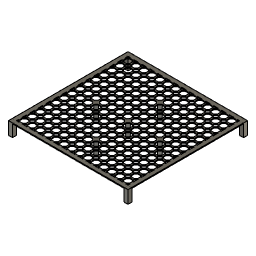
anticoprophagia mouse bedding (Autodesk Fusion 360 design; units mm, degrees)
Autodesk Fusion 360 part; units mm, degrees
(part 1 of 6)
sketch "Sketch1" plane through (0, 0, 0) normal (0, 0, 1) x (1, 0, 0)
  line L0 (-75, -75) -> (75, -75)
  line L1 (75, -75) -> (75, 75)
  line L2 (75, 75) -> (-75, 75)
  line L3 (-75, 75) -> (-75, -75)
  line L4 (-75, -75) -> (75, 75) construction
  line L5 (75, -75) -> (-75, 75) construction
  line L6 (-70, 70) -> (70, 70)
  line L7 (70, 70) -> (70, -70)
  line L8 (70, -70) -> (-70, -70)
  line L9 (-70, -70) -> (-70, 70)
  line L10 (-70, 70) -> (70, -70) construction
  line L11 (70, 70) -> (-70, -70) construction
  line L12 (-70, 70) -> (-60, 70)
  line L13 (-62.9289, 60) -> (-60, 62.9289)
  line L14 (-60, 62.9289) -> (-60, 67.0711)
  line L15 (-60, 67.0711) -> (-62.9289, 70)
  line L16 (-62.9289, 70) -> (-67.0711, 70)
  line L17 (-67.0711, 70) -> (-70, 67.0711)
  line L18 (-70, 67.0711) -> (-70, 62.9289)
  line L19 (-70, 62.9289) -> (-67.0711, 60)
  line L20 (-67.0711, 60) -> (-62.9289, 60)
  line L21 (-61, 63.3431) -> (-61, 66.6569)
  line L22 (-61, 66.6569) -> (-63.3431, 69)
  line L23 (-63.3431, 69) -> (-66.6569, 69)
  line L24 (-66.6569, 69) -> (-69, 66.6569)
  line L25 (-69, 66.6569) -> (-69, 63.3431)
  line L26 (-69, 63.3431) -> (-66.6569, 61)
  line L27 (-66.6569, 61) -> (-63.3431, 61)
  line L28 (-63.3431, 61) -> (-61, 63.3431)
  line L29 (-60, 67.0711) -> (-60, 62.9289)
  line L30 (-57.0711, 70) -> (-60, 67.0711)
  line L31 (-56.6569, 69) -> (-59, 66.6569)
  line L32 (-53.3431, 69) -> (-56.6569, 69)
  line L33 (-51, 66.6569) -> (-53.3431, 69)
  line L34 (-51, 63.3431) -> (-51, 66.6569)
  line L35 (-53.3431, 61) -> (-51, 63.3431)
  line L36 (-56.6569, 61) -> (-53.3431, 61)
  line L37 (-59, 63.3431) -> (-56.6569, 61)
  line L38 (-59, 66.6569) -> (-59, 63.3431)
  line L39 (-60, 62.9289) -> (-57.0711, 60)
  line L40 (-57.0711, 60) -> (-52.9289, 60)
  line L41 (-52.9289, 60) -> (-50, 62.9289)
  line L42 (-50, 62.9289) -> (-50, 67.0711)
  line L43 (-50, 67.0711) -> (-52.9289, 70)
  line L44 (-50, 67.0711) -> (-50, 62.9289)
  line L45 (-47.0711, 70) -> (-50, 67.0711)
  line L46 (-46.6569, 69) -> (-49, 66.6569)
  line L47 (-43.3431, 69) -> (-46.6569, 69)
  line L48 (-41, 66.6569) -> (-43.3431, 69)
  line L49 (-41, 63.3431) -> (-41, 66.6569)
  line L50 (-43.3431, 61) -> (-41, 63.3431)
  line L51 (-46.6569, 61) -> (-43.3431, 61)
  line L52 (-49, 63.3431) -> (-46.6569, 61)
  line L53 (-49, 66.6569) -> (-49, 63.3431)
  line L54 (-50, 62.9289) -> (-47.0711, 60)
  line L55 (-47.0711, 60) -> (-42.9289, 60)
  line L56 (-42.9289, 60) -> (-40, 62.9289)
  line L57 (-40, 62.9289) -> (-40, 67.0711)
  line L58 (-40, 67.0711) -> (-42.9289, 70)
  line L59 (-40, 67.0711) -> (-40, 62.9289)
  line L60 (-37.0711, 70) -> (-40, 67.0711)
  line L61 (-36.6569, 69) -> (-39, 66.6569)
  line L62 (-33.3431, 69) -> (-36.6569, 69)
  line L63 (-31, 66.6569) -> (-33.3431, 69)
  line L64 (-31, 63.3431) -> (-31, 66.6569)
  line L65 (-33.3431, 61) -> (-31, 63.3431)
  line L66 (-36.6569, 61) -> (-33.3431, 61)
  line L67 (-39, 63.3431) -> (-36.6569, 61)
  line L68 (-39, 66.6569) -> (-39, 63.3431)
  line L69 (-40, 62.9289) -> (-37.0711, 60)
  line L70 (-37.0711, 60) -> (-32.9289, 60)
  line L71 (-32.9289, 60) -> (-30, 62.9289)
  line L72 (-30, 62.9289) -> (-30, 67.0711)
  line L73 (-30, 67.0711) -> (-32.9289, 70)
  line L74 (-30, 67.0711) -> (-30, 62.9289)
  line L75 (-27.0711, 70) -> (-30, 67.0711)
  line L76 (-26.6569, 69) -> (-29, 66.6569)
  line L77 (-23.3431, 69) -> (-26.6569, 69)
  line L78 (-21, 66.6569) -> (-23.3431, 69)
  line L79 (-21, 63.3431) -> (-21, 66.6569)
  line L80 (-23.3431, 61) -> (-21, 63.3431)
  line L81 (-26.6569, 61) -> (-23.3431, 61)
  line L82 (-29, 63.3431) -> (-26.6569, 61)
  line L83 (-29, 66.6569) -> (-29, 63.3431)
  line L84 (-30, 62.9289) -> (-27.0711, 60)
  line L85 (-27.0711, 60) -> (-22.9289, 60)
  line L86 (-22.9289, 60) -> (-20, 62.9289)
  line L87 (-20, 62.9289) -> (-20, 67.0711)
  line L88 (-20, 67.0711) -> (-22.9289, 70)
  line L89 (-20, 67.0711) -> (-20, 62.9289)
  line L90 (-17.0711, 70) -> (-20, 67.0711)
  line L91 (-16.6569, 69) -> (-19, 66.6569)
  line L92 (-13.3431, 69) -> (-16.6569, 69)
  line L93 (-11, 66.6569) -> (-13.3431, 69)
  line L94 (-11, 63.3431) -> (-11, 66.6569)
  line L95 (-13.3431, 61) -> (-11, 63.3431)
  line L96 (-16.6569, 61) -> (-13.3431, 61)
  line L97 (-19, 63.3431) -> (-16.6569, 61)
  line L98 (-19, 66.6569) -> (-19, 63.3431)
  line L99 (-20, 62.9289) -> (-17.0711, 60)
  line L100 (-17.0711, 60) -> (-12.9289, 60)
  line L101 (-12.9289, 60) -> (-10, 62.9289)
  line L102 (-10, 62.9289) -> (-10, 67.0711)
  line L103 (-10, 67.0711) -> (-12.9289, 70)
  line L104 (-10, 67.0711) -> (-10, 62.9289)
  line L105 (-7.0711, 70) -> (-10, 67.0711)
  line L106 (-6.6569, 69) -> (-9, 66.6569)
  line L107 (-3.3431, 69) -> (-6.6569, 69)
  line L108 (-1, 66.6569) -> (-3.3431, 69)
  line L109 (-1, 63.3431) -> (-1, 66.6569)
  line L110 (-3.3431, 61) -> (-1, 63.3431)
  line L111 (-6.6569, 61) -> (-3.3431, 61)
  line L112 (-9, 63.3431) -> (-6.6569, 61)
  line L113 (-9, 66.6569) -> (-9, 63.3431)
  line L114 (-10, 62.9289) -> (-7.0711, 60)
  line L115 (-7.0711, 60) -> (-2.9289, 60)
  line L116 (-2.9289, 60) -> (0, 62.9289)
  line L117 (0, 62.9289) -> (0, 67.0711)
  line L118 (0, 67.0711) -> (-2.9289, 70)
  line L119 (0, 67.0711) -> (0, 62.9289)
  line L120 (2.9289, 70) -> (0, 67.0711)
  line L121 (3.3431, 69) -> (1, 66.6569)
  line L122 (6.6569, 69) -> (3.3431, 69)
  line L123 (9, 66.6569) -> (6.6569, 69)
  line L124 (9, 63.3431) -> (9, 66.6569)
  line L125 (6.6569, 61) -> (9, 63.3431)
  line L126 (3.3431, 61) -> (6.6569, 61)
  line L127 (1, 63.3431) -> (3.3431, 61)
  line L128 (1, 66.6569) -> (1, 63.3431)
  line L129 (0, 62.9289) -> (2.9289, 60)
  line L130 (2.9289, 60) -> (7.0711, 60)
  line L131 (7.0711, 60) -> (10, 62.9289)
  line L132 (10, 62.9289) -> (10, 67.0711)
  line L133 (10, 67.0711) -> (7.0711, 70)
  line L134 (10, 67.0711) -> (10, 62.9289)
  line L135 (12.9289, 70) -> (10, 67.0711)
  line L136 (13.3431, 69) -> (11, 66.6569)
  line L137 (16.6569, 69) -> (13.3431, 69)
  line L138 (19, 66.6569) -> (16.6569, 69)
  line L139 (19, 63.3431) -> (19, 66.6569)
  line L140 (16.6569, 61) -> (19, 63.3431)
  line L141 (13.3431, 61) -> (16.6569, 61)
  line L142 (11, 63.3431) -> (13.3431, 61)
  line L143 (11, 66.6569) -> (11, 63.3431)
  line L144 (10, 62.9289) -> (12.9289, 60)
  line L145 (12.9289, 60) -> (17.0711, 60)
  line L146 (17.0711, 60) -> (20, 62.9289)
  line L147 (20, 62.9289) -> (20, 67.0711)
  line L148 (20, 67.0711) -> (17.0711, 70)
  line L149 (20, 67.0711) -> (20, 62.9289)
  line L150 (22.9289, 70) -> (20, 67.0711)
  line L151 (23.3431, 69) -> (21, 66.6569)
  line L152 (26.6569, 69) -> (23.3431, 69)
  line L153 (29, 66.6569) -> (26.6569, 69)
  line L154 (29, 63.3431) -> (29, 66.6569)
  line L155 (26.6569, 61) -> (29, 63.3431)
  line L156 (23.3431, 61) -> (26.6569, 61)
  line L157 (21, 63.3431) -> (23.3431, 61)
  line L158 (21, 66.6569) -> (21, 63.3431)
  line L159 (20, 62.9289) -> (22.9289, 60)
  line L160 (22.9289, 60) -> (27.0711, 60)
  line L161 (27.0711, 60) -> (30, 62.9289)
  line L162 (30, 62.9289) -> (30, 67.0711)
  line L163 (30, 67.0711) -> (27.0711, 70)
  line L164 (30, 67.0711) -> (30, 62.9289)
  line L165 (32.9289, 70) -> (30, 67.0711)
  line L166 (33.3431, 69) -> (31, 66.6569)
  line L167 (36.6569, 69) -> (33.3431, 69)
  line L168 (39, 66.6569) -> (36.6569, 69)
  line L169 (39, 63.3431) -> (39, 66.6569)
  line L170 (36.6569, 61) -> (39, 63.3431)
  line L171 (33.3431, 61) -> (36.6569, 61)
  line L172 (31, 63.3431) -> (33.3431, 61)
  line L173 (31, 66.6569) -> (31, 63.3431)
  line L174 (30, 62.9289) -> (32.9289, 60)
  line L175 (32.9289, 60) -> (37.0711, 60)
  line L176 (37.0711, 60) -> (40, 62.9289)
  line L177 (40, 62.9289) -> (40, 67.0711)
  line L178 (40, 67.0711) -> (37.0711, 70)
  line L179 (40, 67.0711) -> (40, 62.9289)
  line L180 (42.9289, 70) -> (40, 67.0711)
  line L181 (43.3431, 69) -> (41, 66.6569)
  line L182 (46.6569, 69) -> (43.3431, 69)
  line L183 (49, 66.6569) -> (46.6569, 69)
  line L184 (49, 63.3431) -> (49, 66.6569)
  line L185 (46.6569, 61) -> (49, 63.3431)
  line L186 (43.3431, 61) -> (46.6569, 61)
  line L187 (41, 63.3431) -> (43.3431, 61)
  line L188 (41, 66.6569) -> (41, 63.3431)
  line L189 (40, 62.9289) -> (42.9289, 60)
  line L190 (42.9289, 60) -> (47.0711, 60)
  line L191 (47.0711, 60) -> (50, 62.9289)
  line L192 (50, 62.9289) -> (50, 67.0711)
  line L193 (50, 67.0711) -> (47.0711, 70)
  line L194 (50, 67.0711) -> (50, 62.9289)
  line L195 (52.9289, 70) -> (50, 67.0711)
  line L196 (53.3431, 69) -> (51, 66.6569)
  line L197 (56.6569, 69) -> (53.3431, 69)
  line L198 (59, 66.6569) -> (56.6569, 69)
  line L199 (59, 63.3431) -> (59, 66.6569)
  line L200 (56.6569, 61) -> (59, 63.3431)
  line L201 (53.3431, 61) -> (56.6569, 61)
  line L202 (51, 63.3431) -> (53.3431, 61)
  line L203 (51, 66.6569) -> (51, 63.3431)
  line L204 (50, 62.9289) -> (52.9289, 60)
  line L205 (52.9289, 60) -> (57.0711, 60)
  line L206 (57.0711, 60) -> (60, 62.9289)
  line L207 (60, 62.9289) -> (60, 67.0711)
  line L208 (60, 67.0711) -> (57.0711, 70)
  line L209 (60, 67.0711) -> (60, 62.9289)
  line L210 (62.9289, 70) -> (60, 67.0711)
  line L211 (63.3431, 69) -> (61, 66.6569)
  line L212 (66.6569, 69) -> (63.3431, 69)
  line L213 (69, 66.6569) -> (66.6569, 69)
  line L214 (69, 63.3431) -> (69, 66.6569)
  line L215 (66.6569, 61) -> (69, 63.3431)
  line L216 (63.3431, 61) -> (66.6569, 61)
  line L217 (61, 63.3431) -> (63.3431, 61)
  line L218 (61, 66.6569) -> (61, 63.3431)
  line L219 (60, 62.9289) -> (62.9289, 60)
  line L220 (62.9289, 60) -> (67.0711, 60)
  line L221 (67.0711, 60) -> (70, 62.9289)
  line L222 (70, 62.9289) -> (70, 67.0711)
  line L223 (70, 67.0711) -> (67.0711, 70)
  line L224 (-70, 57.0711) -> (-70, 52.9289)
  line L225 (-67.0711, 60) -> (-70, 57.0711)
  line L226 (-66.6569, 59) -> (-69, 56.6569)
  line L227 (-63.3431, 59) -> (-66.6569, 59)
  line L228 (-61, 56.6569) -> (-63.3431, 59)
  line L229 (-61, 53.3431) -> (-61, 56.6569)
  line L230 (-63.3431, 51) -> (-61, 53.3431)
  line L231 (-66.6569, 51) -> (-63.3431, 51)
  line L232 (-69, 53.3431) -> (-66.6569, 51)
  line L233 (-69, 56.6569) -> (-69, 53.3431)
  line L234 (-70, 52.9289) -> (-67.0711, 50)
  line L235 (-67.0711, 50) -> (-62.9289, 50)
  line L236 (-62.9289, 50) -> (-60, 52.9289)
  line L237 (-60, 52.9289) -> (-60, 57.0711)
  line L238 (-60, 57.0711) -> (-62.9289, 60)
  line L239 (-60, 57.0711) -> (-60, 52.9289)
  line L240 (-57.0711, 60) -> (-60, 57.0711)
  line L241 (-56.6569, 59) -> (-59, 56.6569)
  line L242 (-53.3431, 59) -> (-56.6569, 59)
  line L243 (-51, 56.6569) -> (-53.3431, 59)
  line L244 (-51, 53.3431) -> (-51, 56.6569)
  line L245 (-53.3431, 51) -> (-51, 53.3431)
  line L246 (-56.6569, 51) -> (-53.3431, 51)
  line L247 (-59, 53.3431) -> (-56.6569, 51)
  line L248 (-59, 56.6569) -> (-59, 53.3431)
  line L249 (-60, 52.9289) -> (-57.0711, 50)
  line L250 (-57.0711, 50) -> (-52.9289, 50)
  line L251 (-52.9289, 50) -> (-50, 52.9289)
  line L252 (-50, 52.9289) -> (-50, 57.0711)
  line L253 (-50, 57.0711) -> (-52.9289, 60)
  line L254 (-50, 57.0711) -> (-50, 52.9289)
  line L255 (-47.0711, 60) -> (-50, 57.0711)
  line L256 (-46.6569, 59) -> (-49, 56.6569)
  line L257 (-43.3431, 59) -> (-46.6569, 59)
  line L258 (-41, 56.6569) -> (-43.3431, 59)
  line L259 (-41, 53.3431) -> (-41, 56.6569)
  line L260 (-43.3431, 51) -> (-41, 53.3431)
  line L261 (-46.6569, 51) -> (-43.3431, 51)
  line L262 (-49, 53.3431) -> (-46.6569, 51)
  line L263 (-49, 56.6569) -> (-49, 53.3431)
  line L264 (-50, 52.9289) -> (-47.0711, 50)
  line L265 (-47.0711, 50) -> (-42.9289, 50)
  line L266 (-42.9289, 50) -> (-40, 52.9289)
  line L267 (-40, 52.9289) -> (-40, 57.0711)
  line L268 (-40, 57.0711) -> (-42.9289, 60)
  line L269 (-40, 57.0711) -> (-40, 52.9289)
  line L270 (-37.0711, 60) -> (-40, 57.0711)
  line L271 (-36.6569, 59) -> (-39, 56.6569)
  line L272 (-33.3431, 59) -> (-36.6569, 59)
  line L273 (-31, 56.6569) -> (-33.3431, 59)
  line L274 (-31, 53.3431) -> (-31, 56.6569)
  line L275 (-33.3431, 51) -> (-31, 53.3431)
  line L276 (-36.6569, 51) -> (-33.3431, 51)
  line L277 (-39, 53.3431) -> (-36.6569, 51)
  line L278 (-39, 56.6569) -> (-39, 53.3431)
  line L279 (-40, 52.9289) -> (-37.0711, 50)
  line L280 (-37.0711, 50) -> (-32.9289, 50)
  line L281 (-32.9289, 50) -> (-30, 52.9289)
  line L282 (-30, 52.9289) -> (-30, 57.0711)
  line L283 (-30, 57.0711) -> (-32.9289, 60)
  line L284 (-30, 57.0711) -> (-30, 52.9289)
  line L285 (-27.0711, 60) -> (-30, 57.0711)
  line L286 (-26.6569, 59) -> (-29, 56.6569)
  line L287 (-23.3431, 59) -> (-26.6569, 59)
  line L288 (-21, 56.6569) -> (-23.3431, 59)
  line L289 (-21, 53.3431) -> (-21, 56.6569)
  line L290 (-23.3431, 51) -> (-21, 53.3431)
  line L291 (-26.6569, 51) -> (-23.3431, 51)
  line L292 (-29, 53.3431) -> (-26.6569, 51)
  line L293 (-29, 56.6569) -> (-29, 53.3431)
  line L294 (-30, 52.9289) -> (-27.0711, 50)
  line L295 (-27.0711, 50) -> (-22.9289, 50)
  line L296 (-22.9289, 50) -> (-20, 52.9289)
  line L297 (-20, 52.9289) -> (-20, 57.0711)
  line L298 (-20, 57.0711) -> (-22.9289, 60)
  line L299 (-20, 57.0711) -> (-20, 52.9289)
  line L300 (-17.0711, 60) -> (-20, 57.0711)
  line L301 (-16.6569, 59) -> (-19, 56.6569)
  line L302 (-13.3431, 59) -> (-16.6569, 59)
  line L303 (-11, 56.6569) -> (-13.3431, 59)
  line L304 (-11, 53.3431) -> (-11, 56.6569)
  line L305 (-13.3431, 51) -> (-11, 53.3431)
  line L306 (-16.6569, 51) -> (-13.3431, 51)
  line L307 (-19, 53.3431) -> (-16.6569, 51)
  line L308 (-19, 56.6569) -> (-19, 53.3431)
  line L309 (-20, 52.9289) -> (-17.0711, 50)
  line L310 (-17.0711, 50) -> (-12.9289, 50)
  line L311 (-12.9289, 50) -> (-10, 52.9289)
  line L312 (-10, 52.9289) -> (-10, 57.0711)
  line L313 (-10, 57.0711) -> (-12.9289, 60)
  line L314 (-10, 57.0711) -> (-10, 52.9289)
  line L315 (-7.0711, 60) -> (-10, 57.0711)
  line L316 (-6.6569, 59) -> (-9, 56.6569)
  line L317 (-3.3431, 59) -> (-6.6569, 59)
  line L318 (-1, 56.6569) -> (-3.3431, 59)
  line L319 (-1, 53.3431) -> (-1, 56.6569)
  line L320 (-3.3431, 51) -> (-1, 53.3431)
  line L321 (-6.6569, 51) -> (-3.3431, 51)
  line L322 (-9, 53.3431) -> (-6.6569, 51)
  line L323 (-9, 56.6569) -> (-9, 53.3431)
  line L324 (-10, 52.9289) -> (-7.0711, 50)
  line L325 (-7.0711, 50) -> (-2.9289, 50)
  line L326 (-2.9289, 50) -> (0, 52.9289)
  line L327 (0, 52.9289) -> (0, 57.0711)
  line L328 (0, 57.0711) -> (-2.9289, 60)
  line L329 (0, 57.0711) -> (0, 52.9289)
  line L330 (2.9289, 60) -> (0, 57.0711)
  line L331 (3.3431, 59) -> (1, 56.6569)
  line L332 (6.6569, 59) -> (3.3431, 59)
  line L333 (9, 56.6569) -> (6.6569, 59)
  line L334 (9, 53.3431) -> (9, 56.6569)
  line L335 (6.6569, 51) -> (9, 53.3431)
  line L336 (3.3431, 51) -> (6.6569, 51)
  line L337 (1, 53.3431) -> (3.3431, 51)
  line L338 (1, 56.6569) -> (1, 53.3431)
  line L339 (0, 52.9289) -> (2.9289, 50)
  line L340 (2.9289, 50) -> (7.0711, 50)
  line L341 (7.0711, 50) -> (10, 52.9289)
  line L342 (10, 52.9289) -> (10, 57.0711)
  line L343 (10, 57.0711) -> (7.0711, 60)
  line L344 (10, 57.0711) -> (10, 52.9289)
  line L345 (12.9289, 60) -> (10, 57.0711)
  line L346 (13.3431, 59) -> (11, 56.6569)
  line L347 (16.6569, 59) -> (13.3431, 59)
  line L348 (19, 56.6569) -> (16.6569, 59)
  line L349 (19, 53.3431) -> (19, 56.6569)
  line L350 (16.6569, 51) -> (19, 53.3431)
  line L351 (13.3431, 51) -> (16.6569, 51)
  line L352 (11, 53.3431) -> (13.3431, 51)
  line L353 (11, 56.6569) -> (11, 53.3431)
  line L354 (10, 52.9289) -> (12.9289, 50)
  line L355 (12.9289, 50) -> (17.0711, 50)
  line L356 (17.0711, 50) -> (20, 52.9289)
  line L357 (20, 52.9289) -> (20, 57.0711)
  line L358 (20, 57.0711) -> (17.0711, 60)
  line L359 (20, 57.0711) -> (20, 52.9289)
  line L360 (22.9289, 60) -> (20, 57.0711)
  line L361 (23.3431, 59) -> (21, 56.6569)
  line L362 (26.6569, 59) -> (23.3431, 59)
  line L363 (29, 56.6569) -> (26.6569, 59)
  line L364 (29, 53.3431) -> (29, 56.6569)
  line L365 (26.6569, 51) -> (29, 53.3431)
  line L366 (23.3431, 51) -> (26.6569, 51)
  line L367 (21, 53.3431) -> (23.3431, 51)
  line L368 (21, 56.6569) -> (21, 53.3431)
  line L369 (20, 52.9289) -> (22.9289, 50)
  line L370 (22.9289, 50) -> (27.0711, 50)
  line L371 (27.0711, 50) -> (30, 52.9289)
  line L372 (30, 52.9289) -> (30, 57.0711)
  line L373 (30, 57.0711) -> (27.0711, 60)
  line L374 (30, 57.0711) -> (30, 52.9289)
  line L375 (32.9289, 60) -> (30, 57.0711)
  line L376 (33.3431, 59) -> (31, 56.6569)
  line L377 (36.6569, 59) -> (33.3431, 59)
  line L378 (39, 56.6569) -> (36.6569, 59)
  line L379 (39, 53.3431) -> (39, 56.6569)
  line L380 (36.6569, 51) -> (39, 53.3431)
  line L381 (33.3431, 51) -> (36.6569, 51)
  line L382 (31, 53.3431) -> (33.3431, 51)
  line L383 (31, 56.6569) -> (31, 53.3431)
  line L384 (30, 52.9289) -> (32.9289, 50)
  line L385 (32.9289, 50) -> (37.0711, 50)
  line L386 (37.0711, 50) -> (40, 52.9289)
  line L387 (40, 52.9289) -> (40, 57.0711)
  line L388 (40, 57.0711) -> (37.0711, 60)
  line L389 (40, 57.0711) -> (40, 52.9289)
  line L390 (42.9289, 60) -> (40, 57.0711)
  line L391 (43.3431, 59) -> (41, 56.6569)
  line L392 (46.6569, 59) -> (43.3431, 59)
  line L393 (49, 56.6569) -> (46.6569, 59)
  line L394 (49, 53.3431) -> (49, 56.6569)
  line L395 (46.6569, 51) -> (49, 53.3431)
  line L396 (43.3431, 51) -> (46.6569, 51)
  line L397 (41, 53.3431) -> (43.3431, 51)
  line L398 (41, 56.6569) -> (41, 53.3431)
  line L399 (40, 52.9289) -> (42.9289, 50)
  line L400 (42.9289, 50) -> (47.0711, 50)
  line L401 (47.0711, 50) -> (50, 52.9289)
  line L402 (50, 52.9289) -> (50, 57.0711)
  line L403 (50, 57.0711) -> (47.0711, 60)
  line L404 (50, 57.0711) -> (50, 52.9289)
  line L405 (52.9289, 60) -> (50, 57.0711)
  line L406 (53.3431, 59) -> (51, 56.6569)
  line L407 (56.6569, 59) -> (53.3431, 59)
  line L408 (59, 56.6569) -> (56.6569, 59)
  line L409 (59, 53.3431) -> (59, 56.6569)
  line L410 (56.6569, 51) -> (59, 53.3431)
  line L411 (53.3431, 51) -> (56.6569, 51)
  line L412 (51, 53.3431) -> (53.3431, 51)
  line L413 (51, 56.6569) -> (51, 53.3431)
  line L414 (50, 52.9289) -> (52.9289, 50)
  line L415 (52.9289, 50) -> (57.0711, 50)
  line L416 (57.0711, 50) -> (60, 52.9289)
  line L417 (60, 52.9289) -> (60, 57.0711)
  line L418 (60, 57.0711) -> (57.0711, 60)
  line L419 (60, 57.0711) -> (60, 52.9289)
  line L420 (62.9289, 60) -> (60, 57.0711)
  line L421 (63.3431, 59) -> (61, 56.6569)
  line L422 (66.6569, 59) -> (63.3431, 59)
  line L423 (69, 56.6569) -> (66.6569, 59)
  line L424 (69, 53.3431) -> (69, 56.6569)
  line L425 (66.6569, 51) -> (69, 53.3431)
  line L426 (63.3431, 51) -> (66.6569, 51)
  line L427 (61, 53.3431) -> (63.3431, 51)
  line L428 (61, 56.6569) -> (61, 53.3431)
  line L429 (60, 52.9289) -> (62.9289, 50)
  line L430 (62.9289, 50) -> (67.0711, 50)
  line L431 (67.0711, 50) -> (70, 52.9289)
  line L432 (70, 52.9289) -> (70, 57.0711)
  line L433 (70, 57.0711) -> (67.0711, 60)
  line L434 (-70, 47.0711) -> (-70, 42.9289)
  line L435 (-67.0711, 50) -> (-70, 47.0711)
  line L436 (-66.6569, 49) -> (-69, 46.6569)
  line L437 (-63.3431, 49) -> (-66.6569, 49)
  line L438 (-61, 46.6569) -> (-63.3431, 49)
  line L439 (-61, 43.3431) -> (-61, 46.6569)
  line L440 (-63.3431, 41) -> (-61, 43.3431)
  line L441 (-66.6569, 41) -> (-63.3431, 41)
  line L442 (-69, 43.3431) -> (-66.6569, 41)
  line L443 (-69, 46.6569) -> (-69, 43.3431)
  line L444 (-70, 42.9289) -> (-67.0711, 40)
  line L445 (-67.0711, 40) -> (-62.9289, 40)
  line L446 (-62.9289, 40) -> (-60, 42.9289)
  line L447 (-60, 42.9289) -> (-60, 47.0711)
  line L448 (-60, 47.0711) -> (-62.9289, 50)
  line L449 (-60, 47.0711) -> (-60, 42.9289)
  line L450 (-57.0711, 50) -> (-60, 47.0711)
  line L451 (-56.6569, 49) -> (-59, 46.6569)
  line L452 (-53.3431, 49) -> (-56.6569, 49)
  line L453 (-51, 46.6569) -> (-53.3431, 49)
  line L454 (-51, 43.3431) -> (-51, 46.6569)
  line L455 (-53.3431, 41) -> (-51, 43.3431)
  line L456 (-56.6569, 41) -> (-53.3431, 41)
  line L457 (-59, 43.3431) -> (-56.6569, 41)
  line L458 (-59, 46.6569) -> (-59, 43.3431)
  line L459 (-60, 42.9289) -> (-57.0711, 40)
  line L460 (-57.0711, 40) -> (-52.9289, 40)
  line L461 (-52.9289, 40) -> (-50, 42.9289)
  line L462 (-50, 42.9289) -> (-50, 47.0711)
  line L463 (-50, 47.0711) -> (-52.9289, 50)
  line L464 (-50, 47.0711) -> (-50, 42.9289)
  line L465 (-47.0711, 50) -> (-50, 47.0711)
  line L466 (-46.6569, 49) -> (-49, 46.6569)
  line L467 (-43.3431, 49) -> (-46.6569, 49)
  line L468 (-41, 46.6569) -> (-43.3431, 49)
  line L469 (-41, 43.3431) -> (-41, 46.6569)
  line L470 (-43.3431, 41) -> (-41, 43.3431)
  line L471 (-46.6569, 41) -> (-43.3431, 41)
  line L472 (-49, 43.3431) -> (-46.6569, 41)
  line L473 (-49, 46.6569) -> (-49, 43.3431)
  line L474 (-50, 42.9289) -> (-47.0711, 40)
  line L475 (-47.0711, 40) -> (-42.9289, 40)
  line L476 (-42.9289, 40) -> (-40, 42.9289)
  line L477 (-40, 42.9289) -> (-40, 47.0711)
  line L478 (-40, 47.0711) -> (-42.9289, 50)
  line L479 (-40, 47.0711) -> (-40, 42.9289)
  line L480 (-37.0711, 50) -> (-40, 47.0711)
  line L481 (-36.6569, 49) -> (-39, 46.6569)
  line L482 (-33.3431, 49) -> (-36.6569, 49)
  line L483 (-31, 46.6569) -> (-33.3431, 49)
  line L484 (-31, 43.3431) -> (-31, 46.6569)
  line L485 (-33.3431, 41) -> (-31, 43.3431)
  line L486 (-36.6569, 41) -> (-33.3431, 41)
  line L487 (-39, 43.3431) -> (-36.6569, 41)
  line L488 (-39, 46.6569) -> (-39, 43.3431)
  line L489 (-40, 42.9289) -> (-37.0711, 40)
  line L490 (-37.0711, 40) -> (-32.9289, 40)
  line L491 (-32.9289, 40) -> (-30, 42.9289)
  line L492 (-30, 42.9289) -> (-30, 47.0711)
  line L493 (-30, 47.0711) -> (-32.9289, 50)
  line L494 (-30, 47.0711) -> (-30, 42.9289)
  line L495 (-27.0711, 50) -> (-30, 47.0711)
  line L496 (-26.6569, 49) -> (-29, 46.6569)
  line L497 (-23.3431, 49) -> (-26.6569, 49)
  line L498 (-21, 46.6569) -> (-23.3431, 49)
  line L499 (-21, 43.3431) -> (-21, 46.6569)
  line L500 (-23.3431, 41) -> (-21, 43.3431)
  line L501 (-26.6569, 41) -> (-23.3431, 41)
  line L502 (-29, 43.3431) -> (-26.6569, 41)
  line L503 (-29, 46.6569) -> (-29, 43.3431)
  line L504 (-30, 42.9289) -> (-27.0711, 40)
  line L505 (-27.0711, 40) -> (-22.9289, 40)
  line L506 (-22.9289, 40) -> (-20, 42.9289)
  line L507 (-20, 42.9289) -> (-20, 47.0711)
  line L508 (-20, 47.0711) -> (-22.9289, 50)
  line L509 (-20, 47.0711) -> (-20, 42.9289)
  line L510 (-17.0711, 50) -> (-20, 47.0711)
  line L511 (-16.6569, 49) -> (-19, 46.6569)
  line L512 (-13.3431, 49) -> (-16.6569, 49)
  line L513 (-11, 46.6569) -> (-13.3431, 49)
  line L514 (-11, 43.3431) -> (-11, 46.6569)
  line L515 (-13.3431, 41) -> (-11, 43.3431)
  line L516 (-16.6569, 41) -> (-13.3431, 41)
  line L517 (-19, 43.3431) -> (-16.6569, 41)
  line L518 (-19, 46.6569) -> (-19, 43.3431)
  line L519 (-20, 42.9289) -> (-17.0711, 40)
  line L520 (-17.0711, 40) -> (-12.9289, 40)
  line L521 (-12.9289, 40) -> (-10, 42.9289)
  line L522 (-10, 42.9289) -> (-10, 47.0711)
  line L523 (-10, 47.0711) -> (-12.9289, 50)
  line L524 (-10, 47.0711) -> (-10, 42.9289)
  line L525 (-7.0711, 50) -> (-10, 47.0711)
  line L526 (-6.6569, 49) -> (-9, 46.6569)
  line L527 (-3.3431, 49) -> (-6.6569, 49)
  line L528 (-1, 46.6569) -> (-3.3431, 49)
  line L529 (-1, 43.3431) -> (-1, 46.6569)
  line L530 (-3.3431, 41) -> (-1, 43.3431)
  line L531 (-6.6569, 41) -> (-3.3431, 41)
  line L532 (-9, 43.3431) -> (-6.6569, 41)
  line L533 (-9, 46.6569) -> (-9, 43.3431)
  line L534 (-10, 42.9289) -> (-7.0711, 40)
  line L535 (-7.0711, 40) -> (-2.9289, 40)
  line L536 (-2.9289, 40) -> (0, 42.9289)
  line L537 (0, 42.9289) -> (0, 47.0711)
  line L538 (0, 47.0711) -> (-2.9289, 50)
  line L539 (0, 47.0711) -> (0, 42.9289)
  line L540 (2.9289, 50) -> (0, 47.0711)
  line L541 (3.3431, 49) -> (1, 46.6569)
  line L542 (6.6569, 49) -> (3.3431, 49)
  line L543 (9, 46.6569) -> (6.6569, 49)
  line L544 (9, 43.3431) -> (9, 46.6569)
  line L545 (6.6569, 41) -> (9, 43.3431)
  line L546 (3.3431, 41) -> (6.6569, 41)
  line L547 (1, 43.3431) -> (3.3431, 41)
  line L548 (1, 46.6569) -> (1, 43.3431)
  line L549 (0, 42.9289) -> (2.9289, 40)
  line L550 (2.9289, 40) -> (7.0711, 40)
  line L551 (7.0711, 40) -> (10, 42.9289)
  line L552 (10, 42.9289) -> (10, 47.0711)
  line L553 (10, 47.0711) -> (7.0711, 50)
  line L554 (10, 47.0711) -> (10, 42.9289)
  line L555 (12.9289, 50) -> (10, 47.0711)
  line L556 (13.3431, 49) -> (11, 46.6569)
  line L557 (16.6569, 49) -> (13.3431, 49)
  line L558 (19, 46.6569) -> (16.6569, 49)
  line L559 (19, 43.3431) -> (19, 46.6569)
  line L560 (16.6569, 41) -> (19, 43.3431)
  line L561 (13.3431, 41) -> (16.6569, 41)
  line L562 (11, 43.3431) -> (13.3431, 41)
  line L563 (11, 46.6569) -> (11, 43.3431)
  line L564 (10, 42.9289) -> (12.9289, 40)
  line L565 (12.9289, 40) -> (17.0711, 40)
  line L566 (17.0711, 40) -> (20, 42.9289)
  line L567 (20, 42.9289) -> (20, 47.0711)
  line L568 (20, 47.0711) -> (17.0711, 50)
  line L569 (20, 47.0711) -> (20, 42.9289)
  line L570 (22.9289, 50) -> (20, 47.0711)
  line L571 (23.3431, 49) -> (21, 46.6569)
  line L572 (26.6569, 49) -> (23.3431, 49)
  line L573 (29, 46.6569) -> (26.6569, 49)
  line L574 (29, 43.3431) -> (29, 46.6569)
  line L575 (26.6569, 41) -> (29, 43.3431)
  line L576 (23.3431, 41) -> (26.6569, 41)
  line L577 (21, 43.3431) -> (23.3431, 41)
  line L578 (21, 46.6569) -> (21, 43.3431)
  line L579 (20, 42.9289) -> (22.9289, 40)
  line L580 (22.9289, 40) -> (27.0711, 40)
  line L581 (27.0711, 40) -> (30, 42.9289)
  line L582 (30, 42.9289) -> (30, 47.0711)
  line L583 (30, 47.0711) -> (27.0711, 50)
  line L584 (30, 47.0711) -> (30, 42.9289)
  line L585 (32.9289, 50) -> (30, 47.0711)
  line L586 (33.3431, 49) -> (31, 46.6569)
  line L587 (36.6569, 49) -> (33.3431, 49)
  line L588 (39, 46.6569) -> (36.6569, 49)
  line L589 (39, 43.3431) -> (39, 46.6569)
  line L590 (36.6569, 41) -> (39, 43.3431)
  line L591 (33.3431, 41) -> (36.6569, 41)
  line L592 (31, 43.3431) -> (33.3431, 41)
  line L593 (31, 46.6569) -> (31, 43.3431)
  line L594 (30, 42.9289) -> (32.9289, 40)
  line L595 (32.9289, 40) -> (37.0711, 40)
  line L596 (37.0711, 40) -> (40, 42.9289)
  line L597 (40, 42.9289) -> (40, 47.0711)
  line L598 (40, 47.0711) -> (37.0711, 50)
  line L599 (40, 47.0711) -> (40, 42.9289)
  line L600 (42.9289, 50) -> (40, 47.0711)
  line L601 (43.3431, 49) -> (41, 46.6569)
  line L602 (46.6569, 49) -> (43.3431, 49)
  line L603 (49, 46.6569) -> (46.6569, 49)
  line L604 (49, 43.3431) -> (49, 46.6569)
  line L605 (46.6569, 41) -> (49, 43.3431)
  line L606 (43.3431, 41) -> (46.6569, 41)
  line L607 (41, 43.3431) -> (43.3431, 41)
  line L608 (41, 46.6569) -> (41, 43.3431)
  line L609 (40, 42.9289) -> (42.9289, 40)
  line L610 (42.9289, 40) -> (47.0711, 40)
  line L611 (47.0711, 40) -> (50, 42.9289)
  line L612 (50, 42.9289) -> (50, 47.0711)
  line L613 (50, 47.0711) -> (47.0711, 50)
  line L614 (50, 47.0711) -> (50, 42.9289)
  line L615 (52.9289, 50) -> (50, 47.0711)
  line L616 (53.3431, 49) -> (51, 46.6569)
  line L617 (56.6569, 49) -> (53.3431, 49)
  line L618 (59, 46.6569) -> (56.6569, 49)
  line L619 (59, 43.3431) -> (59, 46.6569)
  line L620 (56.6569, 41) -> (59, 43.3431)
  line L621 (53.3431, 41) -> (56.6569, 41)
  line L622 (51, 43.3431) -> (53.3431, 41)
  line L623 (51, 46.6569) -> (51, 43.3431)
  line L624 (50, 42.9289) -> (52.9289, 40)
  line L625 (52.9289, 40) -> (57.0711, 40)
  line L626 (57.0711, 40) -> (60, 42.9289)
  line L627 (60, 42.9289) -> (60, 47.0711)
  line L628 (60, 47.0711) -> (57.0711, 50)
  line L629 (60, 47.0711) -> (60, 42.9289)
  line L630 (62.9289, 50) -> (60, 47.0711)
  line L631 (63.3431, 49) -> (61, 46.6569)
  line L632 (66.6569, 49) -> (63.3431, 49)
  line L633 (69, 46.6569) -> (66.6569, 49)
  line L634 (69, 43.3431) -> (69, 46.6569)
  line L635 (66.6569, 41) -> (69, 43.3431)
  line L636 (63.3431, 41) -> (66.6569, 41)
  line L637 (61, 43.3431) -> (63.3431, 41)
  line L638 (61, 46.6569) -> (61, 43.3431)
  line L639 (60, 42.9289) -> (62.9289, 40)
  line L640 (62.9289, 40) -> (67.0711, 40)
  line L641 (67.0711, 40) -> (70, 42.9289)
  line L642 (70, 42.9289) -> (70, 47.0711)
  line L643 (70, 47.0711) -> (67.0711, 50)
  line L644 (-70, 37.0711) -> (-70, 32.9289)
  line L645 (-67.0711, 40) -> (-70, 37.0711)
  line L646 (-66.6569, 39) -> (-69, 36.6569)
  line L647 (-63.3431, 39) -> (-66.6569, 39)
  line L648 (-61, 36.6569) -> (-63.3431, 39)
  line L649 (-61, 33.3431) -> (-61, 36.6569)
  line L650 (-63.3431, 31) -> (-61, 33.3431)
  line L651 (-66.6569, 31) -> (-63.3431, 31)
  line L652 (-69, 33.3431) -> (-66.6569, 31)
  line L653 (-69, 36.6569) -> (-69, 33.3431)
  line L654 (-70, 32.9289) -> (-67.0711, 30)
  line L655 (-67.0711, 30) -> (-62.9289, 30)
  line L656 (-62.9289, 30) -> (-60, 32.9289)
  line L657 (-60, 32.9289) -> (-60, 37.0711)
  line L658 (-60, 37.0711) -> (-62.9289, 40)
  line L659 (-60, 37.0711) -> (-60, 32.9289)
  line L660 (-57.0711, 40) -> (-60, 37.0711)
  line L661 (-56.6569, 39) -> (-59, 36.6569)
  line L662 (-53.3431, 39) -> (-56.6569, 39)
  line L663 (-51, 36.6569) -> (-53.3431, 39)
  line L664 (-51, 33.3431) -> (-51, 36.6569)
  line L665 (-53.3431, 31) -> (-51, 33.3431)
  line L666 (-56.6569, 31) -> (-53.3431, 31)
  line L667 (-59, 33.3431) -> (-56.6569, 31)
  line L668 (-59, 36.6569) -> (-59, 33.3431)
  line L669 (-60, 32.9289) -> (-57.0711, 30)
  line L670 (-57.0711, 30) -> (-52.9289, 30)
  line L671 (-52.9289, 30) -> (-50, 32.9289)
  line L672 (-50, 32.9289) -> (-50, 37.0711)
  line L673 (-50, 37.0711) -> (-52.9289, 40)
  line L674 (-50, 37.0711) -> (-50, 32.9289)
  line L675 (-47.0711, 40) -> (-50, 37.0711)
  line L676 (-46.6569, 39) -> (-49, 36.6569)
  line L677 (-43.3431, 39) -> (-46.6569, 39)
  line L678 (-41, 36.6569) -> (-43.3431, 39)
  line L679 (-41, 33.3431) -> (-41, 36.6569)
  line L680 (-43.3431, 31) -> (-41, 33.3431)
  line L681 (-46.6569, 31) -> (-43.3431, 31)
  line L682 (-49, 33.3431) -> (-46.6569, 31)
  line L683 (-49, 36.6569) -> (-49, 33.3431)
  line L684 (-50, 32.9289) -> (-47.0711, 30)
  line L685 (-47.0711, 30) -> (-42.9289, 30)
  line L686 (-42.9289, 30) -> (-40, 32.9289)
  line L687 (-40, 32.9289) -> (-40, 37.0711)
  line L688 (-40, 37.0711) -> (-42.9289, 40)
  line L689 (-40, 37.0711) -> (-40, 32.9289)
  line L690 (-37.0711, 40) -> (-40, 37.0711)
  line L691 (-36.6569, 39) -> (-39, 36.6569)
  line L692 (-33.3431, 39) -> (-36.6569, 39)
  line L693 (-31, 36.6569) -> (-33.3431, 39)
  line L694 (-31, 33.3431) -> (-31, 36.6569)
  line L695 (-33.3431, 31) -> (-31, 33.3431)
  line L696 (-36.6569, 31) -> (-33.3431, 31)
  line L697 (-39, 33.3431) -> (-36.6569, 31)
  line L698 (-39, 36.6569) -> (-39, 33.3431)
  line L699 (-40, 32.9289) -> (-37.0711, 30)
  line L700 (-37.0711, 30) -> (-32.9289, 30)
  line L701 (-32.9289, 30) -> (-30, 32.9289)
  line L702 (-30, 32.9289) -> (-30, 37.0711)
  line L703 (-30, 37.0711) -> (-32.9289, 40)
  line L704 (-30, 37.0711) -> (-30, 32.9289)
  line L705 (-27.0711, 40) -> (-30, 37.0711)
  line L706 (-26.6569, 39) -> (-29, 36.6569)
  line L707 (-23.3431, 39) -> (-26.6569, 39)
  line L708 (-21, 36.6569) -> (-23.3431, 39)
  line L709 (-21, 33.3431) -> (-21, 36.6569)
  line L710 (-23.3431, 31) -> (-21, 33.3431)
  line L711 (-26.6569, 31) -> (-23.3431, 31)
  line L712 (-29, 33.3431) -> (-26.6569, 31)
  line L713 (-29, 36.6569) -> (-29, 33.3431)
  line L714 (-30, 32.9289) -> (-27.0711, 30)
  line L715 (-27.0711, 30) -> (-22.9289, 30)
  line L716 (-22.9289, 30) -> (-20, 32.9289)
  line L717 (-20, 32.9289) -> (-20, 37.0711)
  line L718 (-20, 37.0711) -> (-22.9289, 40)
  line L719 (-20, 37.0711) -> (-20, 32.9289)
  line L720 (-17.0711, 40) -> (-20, 37.0711)
  line L721 (-16.6569, 39) -> (-19, 36.6569)
  line L722 (-13.3431, 39) -> (-16.6569, 39)
  line L723 (-11, 36.6569) -> (-13.3431, 39)
  line L724 (-11, 33.3431) -> (-11, 36.6569)
  line L725 (-13.3431, 31) -> (-11, 33.3431)
  line L726 (-16.6569, 31) -> (-13.3431, 31)
  line L727 (-19, 33.3431) -> (-16.6569, 31)
  line L728 (-19, 36.6569) -> (-19, 33.3431)
  line L729 (-20, 32.9289) -> (-17.0711, 30)
  line L730 (-17.0711, 30) -> (-12.9289, 30)
  line L731 (-12.9289, 30) -> (-10, 32.9289)
  line L732 (-10, 32.9289) -> (-10, 37.0711)
  line L733 (-10, 37.0711) -> (-12.9289, 40)
  line L734 (-10, 37.0711) -> (-10, 32.9289)
  line L735 (-7.0711, 40) -> (-10, 37.0711)
  line L736 (-6.6569, 39) -> (-9, 36.6569)
  line L737 (-3.3431, 39) -> (-6.6569, 39)
  line L738 (-1, 36.6569) -> (-3.3431, 39)
  line L739 (-1, 33.3431) -> (-1, 36.6569)
  line L740 (-3.3431, 31) -> (-1, 33.3431)
  line L741 (-6.6569, 31) -> (-3.3431, 31)
  line L742 (-9, 33.3431) -> (-6.6569, 31)
  line L743 (-9, 36.6569) -> (-9, 33.3431)
  line L744 (-10, 32.9289) -> (-7.0711, 30)
  line L745 (-7.0711, 30) -> (-2.9289, 30)
  line L746 (-2.9289, 30) -> (0, 32.9289)
  line L747 (0, 32.9289) -> (0, 37.0711)
  line L748 (0, 37.0711) -> (-2.9289, 40)
  line L749 (0, 37.0711) -> (0, 32.9289)
  line L750 (2.9289, 40) -> (0, 37.0711)
  line L751 (3.3431, 39) -> (1, 36.6569)
  line L752 (6.6569, 39) -> (3.3431, 39)
  line L753 (9, 36.6569) -> (6.6569, 39)
  line L754 (9, 33.3431) -> (9, 36.6569)
  line L755 (6.6569, 31) -> (9, 33.3431)
  line L756 (3.3431, 31) -> (6.6569, 31)
  line L757 (1, 33.3431) -> (3.3431, 31)
  line L758 (1, 36.6569) -> (1, 33.3431)
  line L759 (0, 32.9289) -> (2.9289, 30)
  line L760 (2.9289, 30) -> (7.0711, 30)
  line L761 (7.0711, 30) -> (10, 32.9289)
  line L762 (10, 32.9289) -> (10, 37.0711)
  line L763 (10, 37.0711) -> (7.0711, 40)
  line L764 (10, 37.0711) -> (10, 32.9289)
  line L765 (12.9289, 40) -> (10, 37.0711)
  line L766 (13.3431, 39) -> (11, 36.6569)
  line L767 (16.6569, 39) -> (13.3431, 39)
  line L768 (19, 36.6569) -> (16.6569, 39)
  line L769 (19, 33.3431) -> (19, 36.6569)
  line L770 (16.6569, 31) -> (19, 33.3431)
  line L771 (13.3431, 31) -> (16.6569, 31)
  line L772 (11, 33.3431) -> (13.3431, 31)
  line L773 (11, 36.6569) -> (11, 33.3431)
  line L774 (10, 32.9289) -> (12.9289, 30)
  line L775 (12.9289, 30) -> (17.0711, 30)
  line L776 (17.0711, 30) -> (20, 32.9289)
  line L777 (20, 32.9289) -> (20, 37.0711)
  line L778 (20, 37.0711) -> (17.0711, 40)
  line L779 (20, 37.0711) -> (20, 32.9289)
  line L780 (22.9289, 40) -> (20, 37.0711)
  line L781 (23.3431, 39) -> (21, 36.6569)
  line L782 (26.6569, 39) -> (23.3431, 39)
  line L783 (29, 36.6569) -> (26.6569, 39)
  line L784 (29, 33.3431) -> (29, 36.6569)
  line L785 (26.6569, 31) -> (29, 33.3431)
  line L786 (23.3431, 31) -> (26.6569, 31)
  line L787 (21, 33.3431) -> (23.3431, 31)
  line L788 (21, 36.6569) -> (21, 33.3431)
  line L789 (20, 32.9289) -> (22.9289, 30)
  line L790 (22.9289, 30) -> (27.0711, 30)
  line L791 (27.0711, 30) -> (30, 32.9289)
  line L792 (30, 32.9289) -> (30, 37.0711)
  line L793 (30, 37.0711) -> (27.0711, 40)
  line L794 (30, 37.0711) -> (30, 32.9289)
  line L795 (32.9289, 40) -> (30, 37.0711)
  line L796 (33.3431, 39) -> (31, 36.6569)
  line L797 (36.6569, 39) -> (33.3431, 39)
  line L798 (39, 36.6569) -> (36.6569, 39)
  line L799 (39, 33.3431) -> (39, 36.6569)
  line L800 (36.6569, 31) -> (39, 33.3431)
  line L801 (33.3431, 31) -> (36.6569, 31)
  line L802 (31, 33.3431) -> (33.3431, 31)
  line L803 (31, 36.6569) -> (31, 33.3431)
  line L804 (30, 32.9289) -> (32.9289, 30)
  line L805 (32.9289, 30) -> (37.0711, 30)
  line L806 (37.0711, 30) -> (40, 32.9289)
  line L807 (40, 32.9289) -> (40, 37.0711)
  line L808 (40, 37.0711) -> (37.0711, 40)
  line L809 (40, 37.0711) -> (40, 32.9289)
  line L810 (42.9289, 40) -> (40, 37.0711)
  line L811 (43.3431, 39) -> (41, 36.6569)
  line L812 (46.6569, 39) -> (43.3431, 39)
  line L813 (49, 36.6569) -> (46.6569, 39)
  line L814 (49, 33.3431) -> (49, 36.6569)
  line L815 (46.6569, 31) -> (49, 33.3431)
  line L816 (43.3431, 31) -> (46.6569, 31)
  line L817 (41, 33.3431) -> (43.3431, 31)
  line L818 (41, 36.6569) -> (41, 33.3431)
  line L819 (40, 32.9289) -> (42.9289, 30)
  line L820 (42.9289, 30) -> (47.0711, 30)
  line L821 (47.0711, 30) -> (50, 32.9289)
  line L822 (50, 32.9289) -> (50, 37.0711)
  line L823 (50, 37.0711) -> (47.0711, 40)
  line L824 (50, 37.0711) -> (50, 32.9289)
  line L825 (52.9289, 40) -> (50, 37.0711)
  line L826 (53.3431, 39) -> (51, 36.6569)
  line L827 (56.6569, 39) -> (53.3431, 39)
  line L828 (59, 36.6569) -> (56.6569, 39)
  line L829 (59, 33.3431) -> (59, 36.6569)
  line L830 (56.6569, 31) -> (59, 33.3431)
  line L831 (53.3431, 31) -> (56.6569, 31)
  line L832 (51, 33.3431) -> (53.3431, 31)
  line L833 (51, 36.6569) -> (51, 33.3431)
  line L834 (50, 32.9289) -> (52.9289, 30)
  line L835 (52.9289, 30) -> (57.0711, 30)
  line L836 (57.0711, 30) -> (60, 32.9289)
  line L837 (60, 32.9289) -> (60, 37.0711)
  line L838 (60, 37.0711) -> (57.0711, 40)
  line L839 (60, 37.0711) -> (60, 32.9289)
  line L840 (62.9289, 40) -> (60, 37.0711)
  line L841 (63.3431, 39) -> (61, 36.6569)
  line L842 (66.6569, 39) -> (63.3431, 39)
  line L843 (69, 36.6569) -> (66.6569, 39)
  line L844 (69, 33.3431) -> (69, 36.6569)
  line L845 (66.6569, 31) -> (69, 33.3431)
  line L846 (63.3431, 31) -> (66.6569, 31)
  line L847 (61, 33.3431) -> (63.3431, 31)
  line L848 (61, 36.6569) -> (61, 33.3431)
  line L849 (60, 32.9289) -> (62.9289, 30)
  line L850 (62.9289, 30) -> (67.0711, 30)
  line L851 (67.0711, 30) -> (70, 32.9289)
  line L852 (70, 32.9289) -> (70, 37.0711)
  line L853 (70, 37.0711) -> (67.0711, 40)
  line L854 (-70, 27.0711) -> (-70, 22.9289)
  line L855 (-67.0711, 30) -> (-70, 27.0711)
  line L856 (-66.6569, 29) -> (-69, 26.6569)
  line L857 (-63.3431, 29) -> (-66.6569, 29)
  line L858 (-61, 26.6569) -> (-63.3431, 29)
  line L859 (-61, 23.3431) -> (-61, 26.6569)
  line L860 (-63.3431, 21) -> (-61, 23.3431)
  line L861 (-66.6569, 21) -> (-63.3431, 21)
  line L862 (-69, 23.3431) -> (-66.6569, 21)
  line L863 (-69, 26.6569) -> (-69, 23.3431)
  line L864 (-70, 22.9289) -> (-67.0711, 20)
  line L865 (-67.0711, 20) -> (-62.9289, 20)
  line L866 (-62.9289, 20) -> (-60, 22.9289)
  line L867 (-60, 22.9289) -> (-60, 27.0711)
  line L868 (-60, 27.0711) -> (-62.9289, 30)
  line L869 (-60, 27.0711) -> (-60, 22.9289)
  line L870 (-57.0711, 30) -> (-60, 27.0711)
  line L871 (-56.6569, 29) -> (-59, 26.6569)
  line L872 (-53.3431, 29) -> (-56.6569, 29)
  line L873 (-51, 26.6569) -> (-53.3431, 29)
  line L874 (-51, 23.3431) -> (-51, 26.6569)
  line L875 (-53.3431, 21) -> (-51, 23.3431)
  line L876 (-56.6569, 21) -> (-53.3431, 21)
  line L877 (-59, 23.3431) -> (-56.6569, 21)
  line L878 (-59, 26.6569) -> (-59, 23.3431)
  line L879 (-60, 22.9289) -> (-57.0711, 20)
  line L880 (-57.0711, 20) -> (-52.9289, 20)
  line L881 (-52.9289, 20) -> (-50, 22.9289)
  line L882 (-50, 22.9289) -> (-50, 27.0711)
  line L883 (-50, 27.0711) -> (-52.9289, 30)
  line L884 (-50, 27.0711) -> (-50, 22.9289)
  line L885 (-47.0711, 30) -> (-50, 27.0711)
  line L886 (-46.6569, 29) -> (-49, 26.6569)
  line L887 (-43.3431, 29) -> (-46.6569, 29)
  line L888 (-41, 26.6569) -> (-43.3431, 29)
  line L889 (-41, 23.3431) -> (-41, 26.6569)
  line L890 (-43.3431, 21) -> (-41, 23.3431)
  line L891 (-46.6569, 21) -> (-43.3431, 21)
  line L892 (-49, 23.3431) -> (-46.6569, 21)
  line L893 (-49, 26.6569) -> (-49, 23.3431)
  line L894 (-50, 22.9289) -> (-47.0711, 20)
  line L895 (-47.0711, 20) -> (-42.9289, 20)
  line L896 (-42.9289, 20) -> (-40, 22.9289)
  line L897 (-40, 22.9289) -> (-40, 27.0711)
  line L898 (-40, 27.0711) -> (-42.9289, 30)
  line L899 (-40, 27.0711) -> (-40, 22.9289)
  line L900 (-37.0711, 30) -> (-40, 27.0711)
  line L901 (-36.6569, 29) -> (-39, 26.6569)
  line L902 (-33.3431, 29) -> (-36.6569, 29)
  line L903 (-31, 26.6569) -> (-33.3431, 29)
  line L904 (-31, 23.3431) -> (-31, 26.6569)
  line L905 (-33.3431, 21) -> (-31, 23.3431)
  line L906 (-36.6569, 21) -> (-33.3431, 21)
  line L907 (-39, 23.3431) -> (-36.6569, 21)
  line L908 (-39, 26.6569) -> (-39, 23.3431)
  line L909 (-40, 22.9289) -> (-37.0711, 20)
  line L910 (-37.0711, 20) -> (-32.9289, 20)
  line L911 (-32.9289, 20) -> (-30, 22.9289)
  line L912 (-30, 22.9289) -> (-30, 27.0711)
  line L913 (-30, 27.0711) -> (-32.9289, 30)
  line L914 (-30, 27.0711) -> (-30, 22.9289)
  line L915 (-27.0711, 30) -> (-30, 27.0711)
  line L916 (-26.6569, 29) -> (-29, 26.6569)
  line L917 (-23.3431, 29) -> (-26.6569, 29)
  line L918 (-21, 26.6569) -> (-23.3431, 29)
  line L919 (-21, 23.3431) -> (-21, 26.6569)
  line L920 (-23.3431, 21) -> (-21, 23.3431)
  line L921 (-26.6569, 21) -> (-23.3431, 21)
  line L922 (-29, 23.3431) -> (-26.6569, 21)
  line L923 (-29, 26.6569) -> (-29, 23.3431)
  line L924 (-30, 22.9289) -> (-27.0711, 20)
  line L925 (-27.0711, 20) -> (-22.9289, 20)
  line L926 (-22.9289, 20) -> (-20, 22.9289)
  line L927 (-20, 22.9289) -> (-20, 27.0711)
  line L928 (-20, 27.0711) -> (-22.9289, 30)
  line L929 (-20, 27.0711) -> (-20, 22.9289)
  line L930 (-17.0711, 30) -> (-20, 27.0711)
  line L931 (-16.6569, 29) -> (-19, 26.6569)
  line L932 (-13.3431, 29) -> (-16.6569, 29)
  line L933 (-11, 26.6569) -> (-13.3431, 29)
  line L934 (-11, 23.3431) -> (-11, 26.6569)
  line L935 (-13.3431, 21) -> (-11, 23.3431)
  line L936 (-16.6569, 21) -> (-13.3431, 21)
  line L937 (-19, 23.3431) -> (-16.6569, 21)
  line L938 (-19, 26.6569) -> (-19, 23.3431)
  line L939 (-20, 22.9289) -> (-17.0711, 20)
  line L940 (-17.0711, 20) -> (-12.9289, 20)
  line L941 (-12.9289, 20) -> (-10, 22.9289)
  line L942 (-10, 22.9289) -> (-10, 27.0711)
  line L943 (-10, 27.0711) -> (-12.9289, 30)
  line L944 (-10, 27.0711) -> (-10, 22.9289)
  line L945 (-7.0711, 30) -> (-10, 27.0711)
  line L946 (-6.6569, 29) -> (-9, 26.6569)
  line L947 (-3.3431, 29) -> (-6.6569, 29)
  line L948 (-1, 26.6569) -> (-3.3431, 29)
  line L949 (-1, 23.3431) -> (-1, 26.6569)
  line L950 (-3.3431, 21) -> (-1, 23.3431)
  line L951 (-6.6569, 21) -> (-3.3431, 21)
  line L952 (-9, 23.3431) -> (-6.6569, 21)
  line L953 (-9, 26.6569) -> (-9, 23.3431)
  line L954 (-10, 22.9289) -> (-7.0711, 20)
  line L955 (-7.0711, 20) -> (-2.9289, 20)
  line L956 (-2.9289, 20) -> (0, 22.9289)
  line L957 (0, 22.9289) -> (0, 27.0711)
  line L958 (0, 27.0711) -> (-2.9289, 30)
  line L959 (0, 27.0711) -> (0, 22.9289)
  line L960 (2.9289, 30) -> (0, 27.0711)
  line L961 (3.3431, 29) -> (1, 26.6569)
  line L962 (6.6569, 29) -> (3.3431, 29)
  line L963 (9, 26.6569) -> (6.6569, 29)
  line L964 (9, 23.3431) -> (9, 26.6569)
  line L965 (6.6569, 21) -> (9, 23.3431)
  line L966 (3.3431, 21) -> (6.6569, 21)
  line L967 (1, 23.3431) -> (3.3431, 21)
  line L968 (1, 26.6569) -> (1, 23.3431)
  line L969 (0, 22.9289) -> (2.9289, 20)
  line L970 (2.9289, 20) -> (7.0711, 20)
  line L971 (7.0711, 20) -> (10, 22.9289)
  line L972 (10, 22.9289) -> (10, 27.0711)
  line L973 (10, 27.0711) -> (7.0711, 30)
  line L974 (10, 27.0711) -> (10, 22.9289)
  line L975 (12.9289, 30) -> (10, 27.0711)
  line L976 (13.3431, 29) -> (11, 26.6569)
  line L977 (16.6569, 29) -> (13.3431, 29)
  line L978 (19, 26.6569) -> (16.6569, 29)
  line L979 (19, 23.3431) -> (19, 26.6569)
  line L980 (16.6569, 21) -> (19, 23.3431)
  line L981 (13.3431, 21) -> (16.6569, 21)
  line L982 (11, 23.3431) -> (13.3431, 21)
  line L983 (11, 26.6569) -> (11, 23.3431)
  line L984 (10, 22.9289) -> (12.9289, 20)
  line L985 (12.9289, 20) -> (17.0711, 20)
  line L986 (17.0711, 20) -> (20, 22.9289)
  line L987 (20, 22.9289) -> (20, 27.0711)
  line L988 (20, 27.0711) -> (17.0711, 30)
  line L989 (20, 27.0711) -> (20, 22.9289)
  line L990 (22.9289, 30) -> (20, 27.0711)
  line L991 (23.3431, 29) -> (21, 26.6569)
  line L992 (26.6569, 29) -> (23.3431, 29)
  line L993 (29, 26.6569) -> (26.6569, 29)
  line L994 (29, 23.3431) -> (29, 26.6569)
  line L995 (26.6569, 21) -> (29, 23.3431)
  line L996 (23.3431, 21) -> (26.6569, 21)
  line L997 (21, 23.3431) -> (23.3431, 21)
  line L998 (21, 26.6569) -> (21, 23.3431)
  line L999 (20, 22.9289) -> (22.9289, 20)
  line L1000 (22.9289, 20) -> (27.0711, 20)
  line L1001 (27.0711, 20) -> (30, 22.9289)
  line L1002 (30, 22.9289) -> (30, 27.0711)
  line L1003 (30, 27.0711) -> (27.0711, 30)
  line L1004 (30, 27.0711) -> (30, 22.9289)
  line L1005 (32.9289, 30) -> (30, 27.0711)
  line L1006 (33.3431, 29) -> (31, 26.6569)
  line L1007 (36.6569, 29) -> (33.3431, 29)
  line L1008 (39, 26.6569) -> (36.6569, 29)
  line L1009 (39, 23.3431) -> (39, 26.6569)
  line L1010 (36.6569, 21) -> (39, 23.3431)
  line L1011 (33.3431, 21) -> (36.6569, 21)
  line L1012 (31, 23.3431) -> (33.3431, 21)
  line L1013 (31, 26.6569) -> (31, 23.3431)
  line L1014 (30, 22.9289) -> (32.9289, 20)
  line L1015 (32.9289, 20) -> (37.0711, 20)
  line L1016 (37.0711, 20) -> (40, 22.9289)
  line L1017 (40, 22.9289) -> (40, 27.0711)
  line L1018 (40, 27.0711) -> (37.0711, 30)
  line L1019 (40, 27.0711) -> (40, 22.9289)
  line L1020 (42.9289, 30) -> (40, 27.0711)
  line L1021 (43.3431, 29) -> (41, 26.6569)
  line L1022 (46.6569, 29) -> (43.3431, 29)
  line L1023 (49, 26.6569) -> (46.6569, 29)
  line L1024 (49, 23.3431) -> (49, 26.6569)
  line L1025 (46.6569, 21) -> (49, 23.3431)
  line L1026 (43.3431, 21) -> (46.6569, 21)
  line L1027 (41, 23.3431) -> (43.3431, 21)
  line L1028 (41, 26.6569) -> (41, 23.3431)
  line L1029 (40, 22.9289) -> (42.9289, 20)
  line L1030 (42.9289, 20) -> (47.0711, 20)
  line L1031 (47.0711, 20) -> (50, 22.9289)
  line L1032 (50, 22.9289) -> (50, 27.0711)
  line L1033 (50, 27.0711) -> (47.0711, 30)
  line L1034 (50, 27.0711) -> (50, 22.9289)
  line L1035 (52.9289, 30) -> (50, 27.0711)
  line L1036 (53.3431, 29) -> (51, 26.6569)
  line L1037 (56.6569, 29) -> (53.3431, 29)
  line L1038 (59, 26.6569) -> (56.6569, 29)
  line L1039 (59, 23.3431) -> (59, 26.6569)
  line L1040 (56.6569, 21) -> (59, 23.3431)
  line L1041 (53.3431, 21) -> (56.6569, 21)
  line L1042 (51, 23.3431) -> (53.3431, 21)
  line L1043 (51, 26.6569) -> (51, 23.3431)
  line L1044 (50, 22.9289) -> (52.9289, 20)
  line L1045 (52.9289, 20) -> (57.0711, 20)
  line L1046 (57.0711, 20) -> (60, 22.9289)
  line L1047 (60, 22.9289) -> (60, 27.0711)
  line L1048 (60, 27.0711) -> (57.0711, 30)
  line L1049 (60, 27.0711) -> (60, 22.9289)
  line L1050 (62.9289, 30) -> (60, 27.0711)
  line L1051 (63.3431, 29) -> (61, 26.6569)
  line L1052 (66.6569, 29) -> (63.3431, 29)
  line L1053 (69, 26.6569) -> (66.6569, 29)
  line L1054 (69, 23.3431) -> (69, 26.6569)
  line L1055 (66.6569, 21) -> (69, 23.3431)
  line L1056 (63.3431, 21) -> (66.6569, 21)
  line L1057 (61, 23.3431) -> (63.3431, 21)
  line L1058 (61, 26.6569) -> (61, 23.3431)
  line L1059 (60, 22.9289) -> (62.9289, 20)
  line L1060 (62.9289, 20) -> (67.0711, 20)
  line L1061 (67.0711, 20) -> (70, 22.9289)
  line L1062 (70, 22.9289) -> (70, 27.0711)
  line L1063 (70, 27.0711) -> (67.0711, 30)
  line L1064 (-70, 17.0711) -> (-70, 12.9289)
  line L1065 (-67.0711, 20) -> (-70, 17.0711)
  line L1066 (-66.6569, 19) -> (-69, 16.6569)
  line L1067 (-63.3431, 19) -> (-66.6569, 19)
  line L1068 (-61, 16.6569) -> (-63.3431, 19)
  line L1069 (-61, 13.3431) -> (-61, 16.6569)
  line L1070 (-63.3431, 11) -> (-61, 13.3431)
  line L1071 (-66.6569, 11) -> (-63.3431, 11)
  line L1072 (-69, 13.3431) -> (-66.6569, 11)
  line L1073 (-69, 16.6569) -> (-69, 13.3431)
  line L1074 (-70, 12.9289) -> (-67.0711, 10)
  line L1075 (-67.0711, 10) -> (-62.9289, 10)
  line L1076 (-62.9289, 10) -> (-60, 12.9289)
  line L1077 (-60, 12.9289) -> (-60, 17.0711)
  line L1078 (-60, 17.0711) -> (-62.9289, 20)
  line L1079 (-60, 17.0711) -> (-60, 12.9289)
  line L1080 (-57.0711, 20) -> (-60, 17.0711)
  line L1081 (-56.6569, 19) -> (-59, 16.6569)
  line L1082 (-53.3431, 19) -> (-56.6569, 19)
  line L1083 (-51, 16.6569) -> (-53.3431, 19)
  line L1084 (-51, 13.3431) -> (-51, 16.6569)
  line L1085 (-53.3431, 11) -> (-51, 13.3431)
  line L1086 (-56.6569, 11) -> (-53.3431, 11)
  line L1087 (-59, 13.3431) -> (-56.6569, 11)
  line L1088 (-59, 16.6569) -> (-59, 13.3431)
  line L1089 (-60, 12.9289) -> (-57.0711, 10)
  line L1090 (-57.0711, 10) -> (-52.9289, 10)
  line L1091 (-52.9289, 10) -> (-50, 12.9289)
  line L1092 (-50, 12.9289) -> (-50, 17.0711)
  line L1093 (-50, 17.0711) -> (-52.9289, 20)
  line L1094 (-50, 17.0711) -> (-50, 12.9289)
  line L1095 (-47.0711, 20) -> (-50, 17.0711)
  line L1096 (-46.6569, 19) -> (-49, 16.6569)
  line L1097 (-43.3431, 19) -> (-46.6569, 19)
  line L1098 (-41, 16.6569) -> (-43.3431, 19)
  line L1099 (-41, 13.3431) -> (-41, 16.6569)
  line L1100 (-43.3431, 11) -> (-41, 13.3431)
  line L1101 (-46.6569, 11) -> (-43.3431, 11)
  line L1102 (-49, 13.3431) -> (-46.6569, 11)
  line L1103 (-49, 16.6569) -> (-49, 13.3431)
  line L1104 (-50, 12.9289) -> (-47.0711, 10)
  line L1105 (-47.0711, 10) -> (-42.9289, 10)
  line L1106 (-42.9289, 10) -> (-40, 12.9289)
  line L1107 (-40, 12.9289) -> (-40, 17.0711)
  line L1108 (-40, 17.0711) -> (-42.9289, 20)
  line L1109 (-40, 17.0711) -> (-40, 12.9289)
  line L1110 (-37.0711, 20) -> (-40, 17.0711)
  line L1111 (-36.6569, 19) -> (-39, 16.6569)
  line L1112 (-33.3431, 19) -> (-36.6569, 19)
  line L1113 (-31, 16.6569) -> (-33.3431, 19)
  line L1114 (-31, 13.3431) -> (-31, 16.6569)
  line L1115 (-33.3431, 11) -> (-31, 13.3431)
  line L1116 (-36.6569, 11) -> (-33.3431, 11)
  line L1117 (-39, 13.3431) -> (-36.6569, 11)
  line L1118 (-39, 16.6569) -> (-39, 13.3431)
  line L1119 (-40, 12.9289) -> (-37.0711, 10)
  line L1120 (-37.0711, 10) -> (-32.9289, 10)
  line L1121 (-32.9289, 10) -> (-30, 12.9289)
  line L1122 (-30, 12.9289) -> (-30, 17.0711)
  line L1123 (-30, 17.0711) -> (-32.9289, 20)
  line L1124 (-30, 17.0711) -> (-30, 12.9289)
  line L1125 (-27.0711, 20) -> (-30, 17.0711)
  line L1126 (-26.6569, 19) -> (-29, 16.6569)
  line L1127 (-23.3431, 19) -> (-26.6569, 19)
  line L1128 (-21, 16.6569) -> (-23.3431, 19)
  line L1129 (-21, 13.3431) -> (-21, 16.6569)
  line L1130 (-23.3431, 11) -> (-21, 13.3431)
  line L1131 (-26.6569, 11) -> (-23.3431, 11)
  line L1132 (-29, 13.3431) -> (-26.6569, 11)
  line L1133 (-29, 16.6569) -> (-29, 13.3431)
  line L1134 (-30, 12.9289) -> (-27.0711, 10)